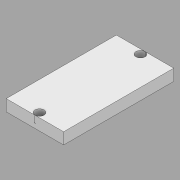
# Autodesk Inventor part: Bottom
Saved by Autodesk Inventor 2019 (Build 230136000, 136)
## iProperties
Created: 2020-02-01
Part Number: Bottom
Material: Generic
Document SubType Name: Modeling
Designer: alb16148
Density: 1 g/cm^3
Appearance: Default
Author: alb16148
Autodesk Inventor part; units mm, degrees
ref_plane "YZ Plane" through (0, 0, 0) normal (1, 0, 0) x (0, 1, 0)
ref_plane "XZ Plane" through (0, 0, 0) normal (0, 1, 0) x (-1, 0, 0)
ref_plane "XY Plane" through (0, 0, 0) normal (0, 0, 1) x (1, 0, 0)
sketch "Sketch1" plane through (0, 0, 0) normal (0, 1, 0) x (-1, 0, 0)
  line L0 (12.5, 24) -> (-12.5, 24)
  line L1 (-12.5, 24) -> (-12.5, -24)
  line L2 (-12.5, -24) -> (12.5, -24)
  line L3 (12.5, -24) -> (12.5, 24)
  point P0 (0, 0)
  dimension "d0" = 12.5
  dimension "d1" = 12.5
  dimension "d2" = 24
  dimension "d3" = 24
  constraints: 8 end point, 2 parallel, 1 horizontal, 1 perpendicular
  measures "d0" distance from line of L3 point (0, 0)
  measures "d1" distance from line of L1 point (0, 0)
  measures "d2" distance from line of L0 point (0, 0)
  measures "d3" distance from line of L2 point (0, 0)
extrude "Extrusion1" add sketch "Sketch1" along normal blind 5
sketch "Sketch2" plane through (0, 5, 0) normal (0, 1, 0) x (1, 0, 0)
  circle A0 centre (0, -22) radius 1.5
  circle A1 centre (0, 22) radius 1.5
  point P0 (0, 0)
  dimension "d6" = 3
  dimension "d7" = 3
  dimension "d8" = 22
  dimension "d9" = 22
  dimension "d10" = 0
  dimension "d11" = 0
  constraints: 2 centre point
  measures "d6" diameter of A0
  measures "d7" diameter of A1
  measures "d8" distance of A0.centre point (0, 0)
  measures "d9" distance of point (0, 0) A1.centre
  measures "d10" horizontal distance of point (0, 0) A0.centre
  measures "d11" horizontal distance of point (0, 0) A1.centre
extrude "Extrusion2" cut sketch "Sketch2" against normal up to surface (5 mm away)
sketch "Sketch4" plane through (0, 5, 0) normal (0, 1, 0) x (1, 0, 0)
  circle A0 centre (0, -22) radius 1.5 projected
  circle A1 centre (0, 22) radius 1.5 projected
  line L0 (-12.5, -24) -> (12.5, -24) projected
  line L1 (12.5, -24) -> (12.5, 24) projected
  line L2 (12.5, 24) -> (-12.5, 24) projected
  line L3 (-12.5, 24) -> (-12.5, -24) projected
  circle A2 centre (0, -22) radius 2
  circle A3 centre (0, 22) radius 2
  point P0 (0, 0)
  dimension "d14" = 4
  dimension "d15" = 4
  constraints: 2 centre point, 2 coincident
  measures "d14" diameter of A2
  measures "d15" diameter of A3
extrude "Extrusion3" cut sketch "Sketch4" against normal blind 3 contours A2 | A3
equation "\"d1\" = d0"
equation "\"d3\" = d2"
body "Solid1"
